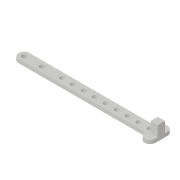
# Autodesk Inventor part: CollectorArm180Final
Saved by Autodesk Inventor 2018 (Build 220112000, 112)
## iProperties
Created: 2018-12-15
Part Number: CollectorArm180Final
Material: Generic
Document SubType Name: Modeling
Designer: ball
Density: 1 g/cm^3
Appearance: Default
Author: ball
Autodesk Inventor part; units mm, degrees
ref_plane "YZ Plane" through (0, 0, 0) normal (1, 0, 0) x (0, 1, 0)
ref_plane "XZ Plane" through (0, 0, 0) normal (0, 1, 0) x (-1, 0, 0)
ref_plane "XY Plane" through (0, 0, 0) normal (0, 0, 1) x (1, 0, 0)
sketch "Sketch1" plane through (0, 0, 0) normal (0, 1, 0) x (-1, 0, 0)
  line L0 (0, 0) -> (22.5655, 0)
  line L1 (22.7982, -9.5222) -> (-0.011, -9.5222)
  line L2 (-0.011, -9.5222) -> (0, 0)
  arc A0 (22.7982, -9.5222) -> (22.5655, 0) centre (20.8435, -4.806) ccw
  line L3 (0, 0) -> (-91.9126, 0)
  line L4 (0, 0) -> (101.4376, 0) construction
  line L5 (-101.4376, 0) -> (-101.4376, -9.525)
  line L6 (0, 0) -> (0, -9.525)
  line L7 (0, -9.525) -> (-91.9126, -9.525)
  circle A1 centre (20.8435, -4.806) radius 2.2479
  line L8 (20.8435, -4.806) -> (4.8415, -4.806) construction
  circle A2 centre (4.8415, -4.806) radius 2.2479
  line L9 (0, -4.7625) -> (-12.7, -4.7625) construction
  circle A3 centre (-12.7, -4.7625) radius 1.9685
  line L10 (0, -4.7625) -> (-101.4376, -4.7625) construction
  circle A4 centre (-22.479, -4.7625) radius 1.9685
  circle A5 centre (-32.258, -4.7625) radius 1.9685
  circle A6 centre (-42.037, -4.7625) radius 1.9685
  circle A7 centre (-51.816, -4.7625) radius 1.9685
  circle A8 centre (-61.595, -4.7625) radius 1.9685
  circle A9 centre (-71.374, -4.7625) radius 1.9685
  circle A10 centre (-81.153, -4.7625) radius 1.9685
  circle A11 centre (-90.932, -4.7625) radius 1.9685
  line L11 (20.8435, -4.806) -> (4.792, -4.806) construction
  line L12 (4.792, -4.806) -> (4.792, 11.196) construction
  line L13 (4.792, 11.196) -> (20.8435, 11.196) construction
  line L14 (20.8435, 11.196) -> (20.8435, -4.806) construction
  line L15 (12.8178, 11.196) -> (12.8178, -4.806) construction
  line L16 (20.8435, 3.195) -> (4.792, 3.195) construction
  circle A12 centre (12.8178, 3.195) radius 1.27 construction
  line L17 (-96.6751, 5.3975) -> (-96.6751, 5.3975)
  line L18 (-96.6751, -14.9225) -> (-96.6751, -14.9225)
  line L19 (-101.4376, -10.16) -> (-101.4376, 0.635)
  arc A13 (-91.9126, 0.635) -> (-96.6751, 5.3975) centre (-96.6751, 0.635) ccw
  arc A14 (-96.6751, 5.3975) -> (-101.4376, 0.635) centre (-96.6751, 0.635) ccw
  arc A15 (-101.4376, -10.16) -> (-96.6751, -14.9225) centre (-96.6751, -10.16) ccw
  arc A16 (-96.6751, -14.9225) -> (-91.9126, -10.16) centre (-96.6751, -10.16) ccw
  line L20 (-91.9126, 0.635) -> (-91.9126, 0)
  line L21 (-91.9126, -9.525) -> (-91.9126, -10.16)
  line L22 (22.7982, -9.5222) -> (22.7982, 0.3175) construction
  point P0 (-91.9126, -14.9225)
  point P1 (-101.4376, -14.9225)
  dimension "d0" = 22.8092
  dimension "d1" = 9.525
  dimension "d2" = 5.1052
  dimension "d4" = 180
  dimension "d7" = 9.525
  dimension "d8" = 9.525
  dimension "d9" = 4.4958
  dimension "d10" = 16.002
  dimension "d11" = 4.4958
  dimension "d12" = 12.7
  dimension "d13" = 3.937
  dimension "d14" = 4.7625
  dimension "d15" = 3.937
  dimension "d16" = 9.779
  dimension "d17" = 3.937
  dimension "d18" = 9.779
  dimension "d19" = 3.937
  dimension "d20" = 9.779
  dimension "d21" = 3.937
  dimension "d22" = 9.779
  dimension "d23" = 3.937
  dimension "d24" = 9.779
  dimension "d25" = 3.937
  dimension "d26" = 9.779
  dimension "d27" = 3.937
  dimension "d28" = 9.779
  dimension "d29" = 3.937
  dimension "d30" = 9.779
  dimension "d31" = 16.002
  dimension "d32" = 2.54
  dimension "d33" = 114.3
  dimension "d36" = 9.525
  dimension "d37" = 10.16
  dimension "d38" = 10.16
  dimension "d39" = 4.7625
  dimension "d44" = 1.9546
  dimension "d45" = 17.5415
  constraints: 44 end point, 17 centre point, 10 point on circle, 10 tangent, 7 midpoint, 6 parallel, 6 perpendicular, 5 horizontal, 3 coincident, 3 equal radius, 3 point on line, 11 other
  measures "d0" distance of L1.start L1.end
  measures "d1" distance of L0.end L1.start
  measures "d2" radius of A0
  measures "d4" angle of L3 L4
  measures "d7" distance of L5.end L5.start
  measures "d8" distance of L0.start L6.end
  measures "d9" diameter of A1
  measures "d10" distance of L8.start L8.end
  measures "d11" diameter of A2
  measures "d12" distance of L9.start L9.end
  measures "d13" diameter of A3
  measures "d14" distance from line of L3 L9.end
  measures "d15" diameter of A4
  measures "d16" distance of A4.centre L9.end
  measures "d17" diameter of A5
  measures "d18" distance of A5.centre A4.centre
  measures "d19" diameter of A6
  measures "d20" distance of A6.centre A5.centre
  measures "d21" diameter of A7
  measures "d22" distance of A7.centre A6.centre
  measures "d23" diameter of A8
  measures "d24" distance of A8.centre A7.centre
  measures "d25" diameter of A9
  measures "d26" distance of A9.centre A8.centre
  measures "d27" diameter of A10
  measures "d28" distance of A10.centre A9.centre
  measures "d29" diameter of A11
  measures "d30" distance of A11.centre A10.centre
  measures "d31" distance of L11.end L12.end
  measures "d32" diameter of A12
  measures "d33" distance of L5.start A12.centre
  measures "d36" distance of point (-91.913, -14.923) point (-101.438, -14.923)
  measures "d39" radius of A13
  measures "d44" distance from line of L22 A0.centre
  measures "d45" horizontal distance of L9.end L8.end
extrude "Extrusion1" add sketch "Sketch1" along normal blind 3.175
sketch "Sketch2" plane through (0, 3.175, 0) normal (0, 1, 0) x (1, 0, 0)
  line L0 (101.4376, -0.635) -> (101.4376, 10.16) construction
  line L1 (95.0876, 4.7625) -> (92.9005, 4.7625) construction
  circle A0 centre (90.932, 4.7625) radius 1.9685 construction
  line L2 (95.0876, 4.7625) -> (95.0876, 7.9375)
  line L3 (95.0876, 7.9375) -> (101.4376, 7.9375)
  line L4 (101.4376, 7.9375) -> (101.4376, 4.7625)
  line L5 (95.0876, 4.7625) -> (95.0876, 1.5875)
  line L6 (95.0876, 1.5875) -> (101.4376, 1.5875)
  line L7 (101.4376, 1.5875) -> (101.4376, 4.7625)
  point P0 (0, 0)
  dimension "d40" = 6.35
  constraints: 14 end point, 2 parallel, 1 horizontal, 1 horizontal alignment, 1 midpoint, 1 point on line, 1 other
  measures "d40" distance of L2.end L3.end
extrude "Extrusion2" add sketch "Sketch2" along normal blind 9.525
body "Solid1"
